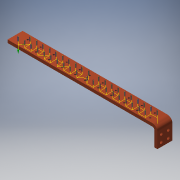
# Autodesk Inventor part: 17-0028-0018
Saved by Autodesk Inventor 2016 SP2 (Build 200236200, 236)
## iProperties
Category: IOP
Company: Universiteit van Amsterdam
RuleStatus: InUse
BeforeDocSave0: Open Form
Created: 2017-11-01
Part Number: 17-0028-0018
Material: Copper
Document SubType Name: Modeling
Designer: Daan Giesen
Density: 8.94 g/cm^3
Appearance: Copper - Satin
Mass: 510.984 g
Surface Area: 268.331 cm^2
Volume: 57.157 cm^3
Project: Digital PID Loop
Cost Center: 17-0028
User Status: CNC
Authority: Reichsöllner, Lukas
Description: Lower bus bar
Author: Daan Giesen
Title: Digital PID Loop
Revision Number: A.1
Autodesk Inventor part; units mm, degrees
ref_plane "YZ Plane" through (0, 0, 0) normal (1, 0, 0) x (0, 1, 0)
ref_plane "XZ Plane" through (0, 0, 0) normal (0, 1, 0) x (-1, 0, 0)
ref_plane "XY Plane" through (0, 0, 0) normal (0, 0, 1) x (1, 0, 0)
sketch "Sketch1" plane through (0, 0, 0) normal (0, 0, 1) x (1, 0, 0)
  line L0 (0, 21) -> (0, -21) construction
  line L1 (-4.2, 0) -> (4.2, 0) construction
  line L2 (-3, -15) -> (3, -15)
  line L3 (3, -15) -> (3, 15)
  line L4 (3, 15) -> (-3, 15)
  line L5 (-3, 15) -> (-3, -15)
  line L6 (-3, -15) -> (3, 15) construction
  line L7 (3, -15) -> (-3, 15) construction
  point P0 (0, 0)
  dimension "d0" = 30
  dimension "d1" = 6
  constraints: 12 end point, 2 midpoint, 2 parallel, 1 horizontal, 1 perpendicular
  measures "d0" distance of L2.end L3.end
  measures "d1" distance of L3.end L4.end
extrude "Extrusion1" add sketch "Sketch1" along normal blind 335
sketch "Sketch2" plane through (3, -15, 0) normal (1, 0, 0) x (0, 0, -1)
  line L0 (0, 0) -> (0, 30) projected
  line L1 (0, 30) -> (-335, 30) projected
  line L2 (-335, 0) -> (-335, 30) projected
  line L3 (0, 0) -> (-335, 0) projected
  line L4 (-30, 0) -> (-30, 30)
  point P0 (0, 15)
  dimension "d4" = 305
  constraints: 2 end point, 2 point on line, 1 perpendicular
  measures "d4" distance between parallel lines of L2 L4
bend part "Bend Part1" radius 10 angle 90 line through (3, -15, 30) along (0, 1, 0) centre toward (-1, 0, 0) moving side (0, 0, 1) both sides no
sketch "Sketch4" plane through (-7, -15, 34) normal (0, 0, -1) x (-1, 0, 0)
  line L0 (25.792, 16.5) -> (25.792, 28) projected
  line L1 (29.992, 16.5) -> (25.792, 16.5) projected
  line L2 (29.992, 11) -> (29.992, 16.5) projected
  line L3 (29.992, 11) -> (17.192, 11) projected
  line L4 (17.192, 11) -> (17.192, 22.5) projected
  line L5 (12.992, 22.5) -> (17.192, 22.5) projected
  line L6 (12.992, 28) -> (12.992, 22.5) projected
  line L7 (12.992, 28) -> (25.792, 28) projected
  arc A0 (15.292, 23.95) -> (15.292, 26.35) centre (15.292, 25.15) ccw projected
  arc A1 (15.292, 26.35) -> (15.292, 23.95) centre (15.292, 25.15) ccw projected
  arc A2 (27.692, 12.65) -> (27.692, 15.05) centre (27.692, 13.85) ccw projected
  arc A3 (27.692, 15.05) -> (27.692, 12.65) centre (27.692, 13.85) ccw projected
  line L8 (38.792, 16.5) -> (38.792, 28) projected
  line L9 (42.992, 16.5) -> (38.792, 16.5) projected
  line L10 (42.992, 11) -> (42.992, 16.5) projected
  line L11 (42.992, 11) -> (30.192, 11) projected
  line L12 (30.192, 11) -> (30.192, 22.5) projected
  line L13 (25.992, 22.5) -> (30.192, 22.5) projected
  line L14 (25.992, 28) -> (25.992, 22.5) projected
  line L15 (25.992, 28) -> (38.792, 28) projected
  arc A4 (28.292, 23.95) -> (28.292, 26.35) centre (28.292, 25.15) ccw projected
  arc A5 (28.292, 26.35) -> (28.292, 23.95) centre (28.292, 25.15) ccw projected
  arc A6 (40.692, 12.65) -> (40.692, 15.05) centre (40.692, 13.85) ccw projected
  arc A7 (40.692, 15.05) -> (40.692, 12.65) centre (40.692, 13.85) ccw projected
  line L16 (51.792, 16.5) -> (51.792, 28) projected
  line L17 (55.992, 16.5) -> (51.792, 16.5) projected
  line L18 (55.992, 11) -> (55.992, 16.5) projected
  line L19 (55.992, 11) -> (43.192, 11) projected
  line L20 (43.192, 11) -> (43.192, 22.5) projected
  line L21 (38.992, 22.5) -> (43.192, 22.5) projected
  line L22 (38.992, 28) -> (38.992, 22.5) projected
  line L23 (38.992, 28) -> (51.792, 28) projected
  arc A8 (41.292, 23.95) -> (41.292, 26.35) centre (41.292, 25.15) ccw projected
  arc A9 (41.292, 26.35) -> (41.292, 23.95) centre (41.292, 25.15) ccw projected
  arc A10 (53.692, 12.65) -> (53.692, 15.05) centre (53.692, 13.85) ccw projected
  arc A11 (53.692, 15.05) -> (53.692, 12.65) centre (53.692, 13.85) ccw projected
  line L24 (64.792, 16.5) -> (64.792, 28) projected
  line L25 (68.992, 16.5) -> (64.792, 16.5) projected
  line L26 (68.992, 11) -> (68.992, 16.5) projected
  line L27 (68.992, 11) -> (56.192, 11) projected
  line L28 (56.192, 11) -> (56.192, 22.5) projected
  line L29 (51.992, 22.5) -> (56.192, 22.5) projected
  line L30 (51.992, 28) -> (51.992, 22.5) projected
  line L31 (51.992, 28) -> (64.792, 28) projected
  arc A12 (54.292, 23.95) -> (54.292, 26.35) centre (54.292, 25.15) ccw projected
  arc A13 (54.292, 26.35) -> (54.292, 23.95) centre (54.292, 25.15) ccw projected
  arc A14 (66.692, 12.65) -> (66.692, 15.05) centre (66.692, 13.85) ccw projected
  arc A15 (66.692, 15.05) -> (66.692, 12.65) centre (66.692, 13.85) ccw projected
  line L32 (77.792, 16.5) -> (77.792, 28) projected
  line L33 (81.992, 16.5) -> (77.792, 16.5) projected
  line L34 (81.992, 11) -> (81.992, 16.5) projected
  line L35 (81.992, 11) -> (69.192, 11) projected
  line L36 (69.192, 11) -> (69.192, 22.5) projected
  line L37 (64.992, 22.5) -> (69.192, 22.5) projected
  line L38 (64.992, 28) -> (64.992, 22.5) projected
  line L39 (64.992, 28) -> (77.792, 28) projected
  arc A16 (67.292, 23.95) -> (67.292, 26.35) centre (67.292, 25.15) ccw projected
  arc A17 (67.292, 26.35) -> (67.292, 23.95) centre (67.292, 25.15) ccw projected
  arc A18 (79.692, 12.65) -> (79.692, 15.05) centre (79.692, 13.85) ccw projected
  arc A19 (79.692, 15.05) -> (79.692, 12.65) centre (79.692, 13.85) ccw projected
  line L40 (90.792, 16.5) -> (90.792, 28) projected
  line L41 (94.992, 16.5) -> (90.792, 16.5) projected
  line L42 (94.992, 11) -> (94.992, 16.5) projected
  line L43 (94.992, 11) -> (82.192, 11) projected
  line L44 (82.192, 11) -> (82.192, 22.5) projected
  line L45 (77.992, 22.5) -> (82.192, 22.5) projected
  line L46 (77.992, 28) -> (77.992, 22.5) projected
  line L47 (77.992, 28) -> (90.792, 28) projected
  arc A20 (80.292, 23.95) -> (80.292, 26.35) centre (80.292, 25.15) ccw projected
  arc A21 (80.292, 26.35) -> (80.292, 23.95) centre (80.292, 25.15) ccw projected
  arc A22 (92.692, 12.65) -> (92.692, 15.05) centre (92.692, 13.85) ccw projected
  arc A23 (92.692, 15.05) -> (92.692, 12.65) centre (92.692, 13.85) ccw projected
  line L48 (103.792, 16.5) -> (103.792, 28) projected
  line L49 (107.992, 16.5) -> (103.792, 16.5) projected
  line L50 (107.992, 11) -> (107.992, 16.5) projected
  line L51 (107.992, 11) -> (95.192, 11) projected
  line L52 (95.192, 11) -> (95.192, 22.5) projected
  line L53 (90.992, 22.5) -> (95.192, 22.5) projected
  line L54 (90.992, 28) -> (90.992, 22.5) projected
  line L55 (90.992, 28) -> (103.792, 28) projected
  arc A24 (93.292, 23.95) -> (93.292, 26.35) centre (93.292, 25.15) ccw projected
  arc A25 (93.292, 26.35) -> (93.292, 23.95) centre (93.292, 25.15) ccw projected
  arc A26 (105.692, 12.65) -> (105.692, 15.05) centre (105.692, 13.85) ccw projected
  arc A27 (105.692, 15.05) -> (105.692, 12.65) centre (105.692, 13.85) ccw projected
  line L56 (116.792, 16.5) -> (116.792, 28) projected
  line L57 (120.992, 16.5) -> (116.792, 16.5) projected
  line L58 (120.992, 11) -> (120.992, 16.5) projected
  line L59 (120.992, 11) -> (108.192, 11) projected
  line L60 (108.192, 11) -> (108.192, 22.5) projected
  line L61 (103.992, 22.5) -> (108.192, 22.5) projected
  line L62 (103.992, 28) -> (103.992, 22.5) projected
  line L63 (103.992, 28) -> (116.792, 28) projected
  arc A28 (106.292, 23.95) -> (106.292, 26.35) centre (106.292, 25.15) ccw projected
  arc A29 (106.292, 26.35) -> (106.292, 23.95) centre (106.292, 25.15) ccw projected
  arc A30 (118.692, 12.65) -> (118.692, 15.05) centre (118.692, 13.85) ccw projected
  arc A31 (118.692, 15.05) -> (118.692, 12.65) centre (118.692, 13.85) ccw projected
  line L64 (129.792, 16.5) -> (129.792, 28) projected
  line L65 (133.992, 16.5) -> (129.792, 16.5) projected
  line L66 (133.992, 11) -> (133.992, 16.5) projected
  line L67 (133.992, 11) -> (121.192, 11) projected
  line L68 (121.192, 11) -> (121.192, 22.5) projected
  line L69 (116.992, 22.5) -> (121.192, 22.5) projected
  line L70 (116.992, 28) -> (116.992, 22.5) projected
  line L71 (116.992, 28) -> (129.792, 28) projected
  arc A32 (119.292, 23.95) -> (119.292, 26.35) centre (119.292, 25.15) ccw projected
  arc A33 (119.292, 26.35) -> (119.292, 23.95) centre (119.292, 25.15) ccw projected
  arc A34 (131.692, 12.65) -> (131.692, 15.05) centre (131.692, 13.85) ccw projected
  arc A35 (131.692, 15.05) -> (131.692, 12.65) centre (131.692, 13.85) ccw projected
  line L72 (142.792, 16.5) -> (142.792, 28) projected
  line L73 (146.992, 16.5) -> (142.792, 16.5) projected
  line L74 (146.992, 11) -> (146.992, 16.5) projected
  line L75 (146.992, 11) -> (134.192, 11) projected
  line L76 (134.192, 11) -> (134.192, 22.5) projected
  line L77 (129.992, 22.5) -> (134.192, 22.5) projected
  line L78 (129.992, 28) -> (129.992, 22.5) projected
  line L79 (129.992, 28) -> (142.792, 28) projected
  arc A36 (132.292, 23.95) -> (132.292, 26.35) centre (132.292, 25.15) ccw projected
  arc A37 (132.292, 26.35) -> (132.292, 23.95) centre (132.292, 25.15) ccw projected
  arc A38 (144.692, 12.65) -> (144.692, 15.05) centre (144.692, 13.85) ccw projected
  arc A39 (144.692, 15.05) -> (144.692, 12.65) centre (144.692, 13.85) ccw projected
  line L80 (163.092, 16.5) -> (163.092, 28) projected
  line L81 (167.292, 16.5) -> (163.092, 16.5) projected
  line L82 (167.292, 11) -> (167.292, 16.5) projected
  line L83 (167.292, 11) -> (154.492, 11) projected
  line L84 (154.492, 11) -> (154.492, 22.5) projected
  line L85 (150.292, 22.5) -> (154.492, 22.5) projected
  line L86 (150.292, 28) -> (150.292, 22.5) projected
  line L87 (150.292, 28) -> (163.092, 28) projected
  arc A40 (152.592, 23.95) -> (152.592, 26.35) centre (152.592, 25.15) ccw projected
  arc A41 (152.592, 26.35) -> (152.592, 23.95) centre (152.592, 25.15) ccw projected
  arc A42 (164.992, 12.65) -> (164.992, 15.05) centre (164.992, 13.85) ccw projected
  arc A43 (164.992, 15.05) -> (164.992, 12.65) centre (164.992, 13.85) ccw projected
  line L88 (176.092, 16.5) -> (176.092, 28) projected
  line L89 (180.292, 16.5) -> (176.092, 16.5) projected
  line L90 (180.292, 11) -> (180.292, 16.5) projected
  line L91 (180.292, 11) -> (167.492, 11) projected
  line L92 (167.492, 11) -> (167.492, 22.5) projected
  line L93 (163.292, 22.5) -> (167.492, 22.5) projected
  line L94 (163.292, 28) -> (163.292, 22.5) projected
  line L95 (163.292, 28) -> (176.092, 28) projected
  arc A44 (165.592, 23.95) -> (165.592, 26.35) centre (165.592, 25.15) ccw projected
  arc A45 (165.592, 26.35) -> (165.592, 23.95) centre (165.592, 25.15) ccw projected
  arc A46 (177.992, 12.65) -> (177.992, 15.05) centre (177.992, 13.85) ccw projected
  arc A47 (177.992, 15.05) -> (177.992, 12.65) centre (177.992, 13.85) ccw projected
  line L96 (189.092, 16.5) -> (189.092, 28) projected
  line L97 (193.292, 16.5) -> (189.092, 16.5) projected
  line L98 (193.292, 11) -> (193.292, 16.5) projected
  line L99 (193.292, 11) -> (180.492, 11) projected
  line L100 (180.492, 11) -> (180.492, 22.5) projected
  line L101 (176.292, 22.5) -> (180.492, 22.5) projected
  line L102 (176.292, 28) -> (176.292, 22.5) projected
  line L103 (176.292, 28) -> (189.092, 28) projected
  arc A48 (178.592, 23.95) -> (178.592, 26.35) centre (178.592, 25.15) ccw projected
  arc A49 (178.592, 26.35) -> (178.592, 23.95) centre (178.592, 25.15) ccw projected
  arc A50 (190.992, 12.65) -> (190.992, 15.05) centre (190.992, 13.85) ccw projected
  arc A51 (190.992, 15.05) -> (190.992, 12.65) centre (190.992, 13.85) ccw projected
  line L104 (202.092, 16.5) -> (202.092, 28) projected
  line L105 (206.292, 16.5) -> (202.092, 16.5) projected
  line L106 (206.292, 11) -> (206.292, 16.5) projected
  line L107 (206.292, 11) -> (193.492, 11) projected
  line L108 (193.492, 11) -> (193.492, 22.5) projected
  line L109 (189.292, 22.5) -> (193.492, 22.5) projected
  line L110 (189.292, 28) -> (189.292, 22.5) projected
  line L111 (189.292, 28) -> (202.092, 28) projected
  arc A52 (191.592, 23.95) -> (191.592, 26.35) centre (191.592, 25.15) ccw projected
  arc A53 (191.592, 26.35) -> (191.592, 23.95) centre (191.592, 25.15) ccw projected
  arc A54 (203.992, 12.65) -> (203.992, 15.05) centre (203.992, 13.85) ccw projected
  arc A55 (203.992, 15.05) -> (203.992, 12.65) centre (203.992, 13.85) ccw projected
  line L112 (215.092, 16.5) -> (215.092, 28) projected
  line L113 (219.292, 16.5) -> (215.092, 16.5) projected
  line L114 (219.292, 11) -> (219.292, 16.5) projected
  line L115 (219.292, 11) -> (206.492, 11) projected
  line L116 (206.492, 11) -> (206.492, 22.5) projected
  line L117 (202.292, 22.5) -> (206.492, 22.5) projected
  line L118 (202.292, 28) -> (202.292, 22.5) projected
  line L119 (202.292, 28) -> (215.092, 28) projected
  arc A56 (204.592, 23.95) -> (204.592, 26.35) centre (204.592, 25.15) ccw projected
  arc A57 (204.592, 26.35) -> (204.592, 23.95) centre (204.592, 25.15) ccw projected
  arc A58 (216.992, 12.65) -> (216.992, 15.05) centre (216.992, 13.85) ccw projected
  arc A59 (216.992, 15.05) -> (216.992, 12.65) centre (216.992, 13.85) ccw projected
  line L120 (228.092, 16.5) -> (228.092, 28) projected
  line L121 (232.292, 16.5) -> (228.092, 16.5) projected
  line L122 (232.292, 11) -> (232.292, 16.5) projected
  line L123 (232.292, 11) -> (219.492, 11) projected
  line L124 (219.492, 11) -> (219.492, 22.5) projected
  line L125 (215.292, 22.5) -> (219.492, 22.5) projected
  line L126 (215.292, 28) -> (215.292, 22.5) projected
  line L127 (215.292, 28) -> (228.092, 28) projected
  arc A60 (217.592, 23.95) -> (217.592, 26.35) centre (217.592, 25.15) ccw projected
  arc A61 (217.592, 26.35) -> (217.592, 23.95) centre (217.592, 25.15) ccw projected
  arc A62 (229.992, 12.65) -> (229.992, 15.05) centre (229.992, 13.85) ccw projected
  arc A63 (229.992, 15.05) -> (229.992, 12.65) centre (229.992, 13.85) ccw projected
  line L128 (241.092, 16.5) -> (241.092, 28) projected
  line L129 (245.292, 16.5) -> (241.092, 16.5) projected
  line L130 (245.292, 11) -> (245.292, 16.5) projected
  line L131 (245.292, 11) -> (232.492, 11) projected
  line L132 (232.492, 11) -> (232.492, 22.5) projected
  line L133 (228.292, 22.5) -> (232.492, 22.5) projected
  line L134 (228.292, 28) -> (228.292, 22.5) projected
  line L135 (228.292, 28) -> (241.092, 28) projected
  arc A64 (230.592, 23.95) -> (230.592, 26.35) centre (230.592, 25.15) ccw projected
  arc A65 (230.592, 26.35) -> (230.592, 23.95) centre (230.592, 25.15) ccw projected
  arc A66 (242.992, 12.65) -> (242.992, 15.05) centre (242.992, 13.85) ccw projected
  arc A67 (242.992, 15.05) -> (242.992, 12.65) centre (242.992, 13.85) ccw projected
  line L136 (254.092, 16.5) -> (254.092, 28) projected
  line L137 (258.292, 16.5) -> (254.092, 16.5) projected
  line L138 (258.292, 11) -> (258.292, 16.5) projected
  line L139 (258.292, 11) -> (245.492, 11) projected
  line L140 (245.492, 11) -> (245.492, 22.5) projected
  line L141 (241.292, 22.5) -> (245.492, 22.5) projected
  line L142 (241.292, 28) -> (241.292, 22.5) projected
  line L143 (241.292, 28) -> (254.092, 28) projected
  arc A68 (243.592, 23.95) -> (243.592, 26.35) centre (243.592, 25.15) ccw projected
  arc A69 (243.592, 26.35) -> (243.592, 23.95) centre (243.592, 25.15) ccw projected
  arc A70 (255.992, 12.65) -> (255.992, 15.05) centre (255.992, 13.85) ccw projected
  arc A71 (255.992, 15.05) -> (255.992, 12.65) centre (255.992, 13.85) ccw projected
  line L144 (267.092, 16.5) -> (267.092, 28) projected
  line L145 (271.292, 16.5) -> (267.092, 16.5) projected
  line L146 (271.292, 11) -> (271.292, 16.5) projected
  line L147 (271.292, 11) -> (258.492, 11) projected
  line L148 (258.492, 11) -> (258.492, 22.5) projected
  line L149 (254.292, 22.5) -> (258.492, 22.5) projected
  line L150 (254.292, 28) -> (254.292, 22.5) projected
  line L151 (254.292, 28) -> (267.092, 28) projected
  arc A72 (256.592, 23.95) -> (256.592, 26.35) centre (256.592, 25.15) ccw projected
  arc A73 (256.592, 26.35) -> (256.592, 23.95) centre (256.592, 25.15) ccw projected
  arc A74 (268.992, 12.65) -> (268.992, 15.05) centre (268.992, 13.85) ccw projected
  arc A75 (268.992, 15.05) -> (268.992, 12.65) centre (268.992, 13.85) ccw projected
  line L152 (280.092, 16.5) -> (280.092, 28) projected
  line L153 (284.292, 16.5) -> (280.092, 16.5) projected
  line L154 (284.292, 11) -> (284.292, 16.5) projected
  line L155 (284.292, 11) -> (271.492, 11) projected
  line L156 (271.492, 11) -> (271.492, 22.5) projected
  line L157 (267.292, 22.5) -> (271.492, 22.5) projected
  line L158 (267.292, 28) -> (267.292, 22.5) projected
  line L159 (267.292, 28) -> (280.092, 28) projected
  arc A76 (269.592, 23.95) -> (269.592, 26.35) centre (269.592, 25.15) ccw projected
  arc A77 (269.592, 26.35) -> (269.592, 23.95) centre (269.592, 25.15) ccw projected
  arc A78 (281.992, 12.65) -> (281.992, 15.05) centre (281.992, 13.85) ccw projected
  arc A79 (281.992, 15.05) -> (281.992, 12.65) centre (281.992, 13.85) ccw projected
  point P0 (-7, 15)
  constraints: 40 coincident
hole "Hole1" at (-22.292, 10.15, 34) at (-34.692, -1.15, 34) at (-35.292, 10.15, 34) at (-48.292, 10.15, 34) at (-47.692, -1.15, 34) at (-60.692, -1.15, 34) at (-61.292, 10.15, 34) at (-74.292, 10.15, 34) at (-73.692, -1.15, 34) at (-86.692, -1.15, 34) at (-87.292, 10.15, 34) at (-100.292, 10.15, 34) at (-99.692, -1.15, 34) at (-113.292, 10.15, 34) at (-112.692, -1.15, 34) at (-126.292, 10.15, 34) at (-125.692, -1.15, 34) at (-139.292, 10.15, 34) at (-138.692, -1.15, 34) at (-151.692, -1.15, 34) at (-159.592, 10.15, 34) at (-172.592, 10.15, 34) at (-171.992, -1.15, 34) at (-185.592, 10.15, 34) at (-184.992, -1.15, 34) at (-198.592, 10.15, 34) at (-197.992, -1.15, 34) at (-211.592, 10.15, 34) at (-210.992, -1.15, 34) at (-224.592, 10.15, 34) at (-223.992, -1.15, 34) at (-237.592, 10.15, 34) at (-236.992, -1.15, 34) at (-250.592, 10.15, 34) at (-249.992, -1.15, 34) at (-263.592, 10.15, 34) at (-262.992, -1.15, 34) at (-276.592, 10.15, 34) at (-275.992, -1.15, 34) at (-288.992, -1.15, 34) direction (0, 0, 1) diameter 1.567 end through all thread size "M2x0.4" class "6H" standard "ISO Metric profile"
sketch "Sketch5" plane through (-296.292, 15, 40) normal (0, 0, 1) x (1, 0, 0)
  line L0 (289.292, -30) -> (0, -30) projected
  line L1 (289.292, 0) -> (0, 0) projected
  line L2 (284, -30) -> (284, 45) projected
  point P0 (296.292, -15)
  point P1 (274.3, -10)
  point P2 (278, -23)
  dimension "d14" = 7
  dimension "d15" = 10
  dimension "d16" = 9.7
  dimension "d17" = 6
  measures "d14" distance from line of point (278, -23) L0
  measures "d15" distance from line of L1 point (274.3, -10)
  measures "d16" distance from line of point (274.3, -10) L2
  measures "d17" distance from line of L2 point (278, -23)
hole "Hole2" at (-21.992, 5, 40) at (-18.292, -8, 40) direction (0, 0, -1) diameter 3.242 end through all thread size "M4x0.7" class "6H" standard "ISO Metric profile"
pattern_linear "Rectangular Pattern1" count 6 spacing 26 along (-1, 0, 0) of "Hole2"
pattern_linear "Rectangular Pattern2" count 2 spacing 150 along (-1, 0, 0) of "Hole2", "Rectangular Pattern1"
sketch "Sketch9" plane through (-3, -15, 30) normal (-1, 0, 0) x (0, 0, 1)
  line L0 (-8, 8) -> (-22, 8) construction
  line L1 (-22, 8) -> (-22, 22) construction
  line L2 (-22, 22) -> (-8, 22) construction
  line L3 (-8, 22) -> (-8, 8) construction
  line L4 (-8, 8) -> (-22, 22) construction
  line L5 (-22, 8) -> (-8, 22) construction
  line L6 (-30, 0) -> (0, 0) projected
  line L7 (-30, 30) -> (-30, 0) projected
  point P0 (-15, 15)
  dimension "d52" = 14
  dimension "d53" = 14
  dimension "d56" = 15
  dimension "d57" = 15
  constraints: 12 end point, 3 coincident, 2 midpoint, 2 parallel, 1 horizontal, 1 perpendicular
  measures "d52" distance of L0.end L1.end
  measures "d53" distance of L1.end L2.end
  measures "d56" distance from line of point (-15, 15) L6
  measures "d57" distance from line of point (-15, 15) L7
hole "Hole4" at (-3, -7, 8) at (-3, -7, 22) at (-3, 7, 22) at (-3, 7, 8) direction (1, 0, 0) diameter 5.3 end through all
sketch "Sketch10" plane through (-7, -15, 34) normal (0, 0, -1) x (-1, 0, 0)
  line L0 (0, 0) -> (289.292, 0) projected
  circle A0 centre (11.292, 7) radius 1.621 projected
  point P0 (-7, 15)
  point P1 (19.892, 6)
  dimension "d78" = 6
  dimension "d79" = 8.6
  measures "d78" distance from line of point (19.892, 6) L0
  measures "d79" horizontal distance of point (19.892, 6) A0.centre
hole "Hole5" at (-26.892, -9, 34) direction (0, 0, 1) diameter 1.8 depth 4 tip angle 118
pattern_linear "Rectangular Pattern4" count 10 spacing 13 along (-1, 0, 0) of "Hole5"
pattern_linear "Rectangular Pattern5" count 2 spacing 137.3 along (-1, 0, 0) of "Hole5", "Rectangular Pattern4"
body "Solid1"
